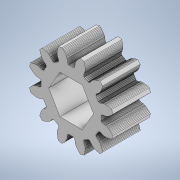
# Autodesk Inventor part: Engranajes_12
Saved by Autodesk Inventor 2022 (Build 260153000, 153)
## iProperties
Created: 2022-02-21
Part Number: Engranajes_12
Material: Generic
Document SubType Name: Modeling
Designer: katha
Density: 1 g/cm^3
Appearance: Default
Author: katha
Autodesk Inventor part; units mm, degrees
(part 1 of 6)
ref_plane "YZ Plane" through (0, 0, 0) normal (1, 0, 0) x (0, 1, 0)
ref_plane "XZ Plane" through (0, 0, 0) normal (0, 1, 0) x (-1, 0, 0)
ref_plane "XY Plane" through (0, 0, 0) normal (0, 0, 1) x (1, 0, 0)
sketch "Sketch1" plane through (0, 0, 0) normal (0, 0, 1) x (1, 0, 0)
  circle A0 centre (36, 0) radius 2
  circle A1 centre (0, 0) radius 2
  circle A2 centre (36, 0) radius 2
  circle A3 centre (0, 0) radius 2
  line L0 (30.8694, -4.5708) -> (30.9098, -4.4161)
  line L1 (30.9098, -4.4161) -> (30.9538, -4.2725)
  line L2 (30.9538, -4.2725) -> (31.0003, -4.1408)
  line L3 (31.0003, -4.1408) -> (31.0488, -4.0198)
  line L4 (31.0488, -4.0198) -> (31.0977, -3.9112)
  line L5 (31.0977, -3.9112) -> (31.1475, -3.8119)
  line L6 (31.1475, -3.8119) -> (31.1956, -3.7252)
  line L7 (31.1956, -3.7252) -> (31.2429, -3.6478)
  line L8 (31.2429, -3.6478) -> (31.2875, -3.5813)
  line L9 (31.2875, -3.5813) -> (31.3671, -3.477)
  line L10 (31.3671, -3.477) -> (31.4285, -3.4089)
  line L11 (31.4285, -3.4089) -> (31.466, -3.3746)
  line L12 (31.466, -3.3746) -> (31.5668, -3.3141)
  line L13 (31.5668, -3.3141) -> (31.6547, -3.2516)
  line L14 (31.6547, -3.2516) -> (31.7296, -3.1879)
  line L15 (31.7296, -3.1879) -> (31.7917, -3.1241)
  line L16 (31.7917, -3.1241) -> (31.841, -3.0611)
  line L17 (31.841, -3.0611) -> (31.8779, -2.9999)
  line L18 (31.8779, -2.9999) -> (31.9025, -2.9414)
  line L19 (31.9025, -2.9414) -> (31.9152, -2.8864)
  line L20 (31.9152, -2.8864) -> (31.9163, -2.836)
  line L21 (31.9163, -2.836) -> (31.9062, -2.7909)
  line L22 (31.9062, -2.7909) -> (31.8916, -2.7611)
  line L23 (31.8916, -2.7611) -> (31.8003, -2.6202)
  line L24 (31.8003, -2.6202) -> (31.7132, -2.475)
  line L25 (31.7132, -2.475) -> (31.631, -2.327)
  line L26 (31.631, -2.327) -> (31.5546, -2.1774)
  line L27 (31.5546, -2.1774) -> (31.5361, -2.1499)
  line L28 (31.5361, -2.1499) -> (31.5021, -2.1186)
  line L29 (31.5021, -2.1186) -> (31.4579, -2.0943)
  line L30 (31.4579, -2.0943) -> (31.404, -2.0778)
  line L31 (31.404, -2.0778) -> (31.341, -2.0699)
  line L32 (31.341, -2.0699) -> (31.2695, -2.0712)
  line L33 (31.2695, -2.0712) -> (31.1903, -2.0825)
  line L34 (31.1903, -2.0825) -> (31.104, -2.1043)
  line L35 (31.104, -2.1043) -> (31.0114, -2.1374)
  line L36 (31.0114, -2.1374) -> (30.9133, -2.1822)
  line L37 (30.9133, -2.1822) -> (30.8106, -2.2393)
  line L38 (30.8106, -2.2393) -> (30.762, -2.2546)
  line L39 (30.762, -2.2546) -> (30.6724, -2.2738)
  line L40 (30.6724, -2.2738) -> (30.5422, -2.2905)
  line L41 (30.5422, -2.2905) -> (30.4624, -2.2959)
  line L42 (30.4624, -2.2959) -> (30.3717, -2.2981)
  line L43 (30.3717, -2.2981) -> (30.2725, -2.2965)
  line L44 (30.2725, -2.2965) -> (30.1616, -2.2899)
  line L45 (30.1616, -2.2899) -> (30.0431, -2.278)
  line L46 (30.0431, -2.278) -> (29.9141, -2.2595)
  line L47 (29.9141, -2.2595) -> (29.7768, -2.2339)
  line L48 (29.7768, -2.2339) -> (29.6305, -2.2002)
  line L49 (29.6305, -2.2002) -> (29.4762, -2.1578)
  line L50 (29.4762, -2.1578) -> (29.3255, -2.1096)
  arc A4 (29.1649, -1.5103) -> (29.3255, -2.1096) centre (36, 0) ccw
  line L51 (29.1649, -1.5103) -> (29.2713, -1.3932)
  line L52 (29.2713, -1.3932) -> (29.3837, -1.2793)
  line L53 (29.3837, -1.2793) -> (29.4936, -1.177)
  line L54 (29.4936, -1.177) -> (29.5997, -1.0861)
  line L55 (29.5997, -1.0861) -> (29.7022, -1.0056)
  line L56 (29.7022, -1.0056) -> (29.7988, -0.9361)
  line L57 (29.7988, -0.9361) -> (29.8916, -0.875)
  line L58 (29.8916, -0.875) -> (29.9767, -0.8239)
  line L59 (29.9767, -0.8239) -> (30.0563, -0.7805)
  line L60 (30.0563, -0.7805) -> (30.1282, -0.7452)
  line L61 (30.1282, -0.7452) -> (30.2493, -0.6947)
  line L62 (30.2493, -0.6947) -> (30.3365, -0.6665)
  line L63 (30.3365, -0.6665) -> (30.3862, -0.6555)
  line L64 (30.3862, -0.6555) -> (30.5037, -0.6535)
  line L65 (30.5037, -0.6535) -> (30.611, -0.6433)
  line L66 (30.611, -0.6433) -> (30.7078, -0.6256)
  line L67 (30.7078, -0.6256) -> (30.7934, -0.6014)
  line L68 (30.7934, -0.6014) -> (30.8677, -0.5716)
  line L69 (30.8677, -0.5716) -> (30.9302, -0.537)
  line L70 (30.9302, -0.537) -> (30.9808, -0.4986)
  line L71 (30.9808, -0.4986) -> (31.0192, -0.4573)
  line L72 (31.0192, -0.4573) -> (31.0454, -0.4142)
  line L73 (31.0454, -0.4142) -> (31.0592, -0.3701)
  line L74 (31.0592, -0.3701) -> (31.0614, -0.337)
  line L75 (31.0614, -0.337) -> (31.0529, -0.1693)
  line L76 (31.0529, -0.1693) -> (31.05, 0)
  line L77 (31.05, 0) -> (31.0529, 0.1693)
  line L78 (31.0529, 0.1693) -> (31.0614, 0.337)
  line L79 (31.0614, 0.337) -> (31.0592, 0.3701)
  line L80 (31.0592, 0.3701) -> (31.0454, 0.4142)
  line L81 (31.0454, 0.4142) -> (31.0192, 0.4573)
  line L82 (31.0192, 0.4573) -> (30.9808, 0.4986)
  line L83 (30.9808, 0.4986) -> (30.9302, 0.537)
  line L84 (30.9302, 0.537) -> (30.8677, 0.5716)
  line L85 (30.8677, 0.5716) -> (30.7934, 0.6014)
  line L86 (30.7934, 0.6014) -> (30.7078, 0.6256)
  line L87 (30.7078, 0.6256) -> (30.611, 0.6433)
  line L88 (30.611, 0.6433) -> (30.5037, 0.6535)
  line L89 (30.5037, 0.6535) -> (30.3862, 0.6555)
  line L90 (30.3862, 0.6555) -> (30.3365, 0.6665)
  line L91 (30.3365, 0.6665) -> (30.2493, 0.6947)
  line L92 (30.2493, 0.6947) -> (30.1282, 0.7452)
  line L93 (30.1282, 0.7452) -> (30.0563, 0.7805)
  line L94 (30.0563, 0.7805) -> (29.9767, 0.8239)
  line L95 (29.9767, 0.8239) -> (29.8916, 0.875)
  line L96 (29.8916, 0.875) -> (29.7988, 0.9361)
  line L97 (29.7988, 0.9361) -> (29.7022, 1.0056)
  line L98 (29.7022, 1.0056) -> (29.5997, 1.0861)
  line L99 (29.5997, 1.0861) -> (29.4936, 1.177)
  line L100 (29.4936, 1.177) -> (29.3837, 1.2793)
  line L101 (29.3837, 1.2793) -> (29.2713, 1.3932)
  line L102 (29.2713, 1.3932) -> (29.1649, 1.5103)
  arc A5 (29.3255, 2.1096) -> (29.1649, 1.5103) centre (36, 0) ccw
  line L103 (29.3255, 2.1096) -> (29.4762, 2.1578)
  line L104 (29.4762, 2.1578) -> (29.6305, 2.2002)
  line L105 (29.6305, 2.2002) -> (29.7768, 2.2339)
  line L106 (29.7768, 2.2339) -> (29.9141, 2.2595)
  line L107 (29.9141, 2.2595) -> (30.0431, 2.278)
  line L108 (30.0431, 2.278) -> (30.1616, 2.2899)
  line L109 (30.1616, 2.2899) -> (30.2725, 2.2965)
  line L110 (30.2725, 2.2965) -> (30.3717, 2.2981)
  line L111 (30.3717, 2.2981) -> (30.4624, 2.2959)
  line L112 (30.4624, 2.2959) -> (30.5422, 2.2905)
  line L113 (30.5422, 2.2905) -> (30.6724, 2.2738)
  line L114 (30.6724, 2.2738) -> (30.762, 2.2546)
  line L115 (30.762, 2.2546) -> (30.8106, 2.2393)
  line L116 (30.8106, 2.2393) -> (30.9133, 2.1822)
  line L117 (30.9133, 2.1822) -> (31.0114, 2.1374)
  line L118 (31.0114, 2.1374) -> (31.104, 2.1043)
  line L119 (31.104, 2.1043) -> (31.1903, 2.0825)
  line L120 (31.1903, 2.0825) -> (31.2695, 2.0712)
  line L121 (31.2695, 2.0712) -> (31.341, 2.0699)
  line L122 (31.341, 2.0699) -> (31.404, 2.0778)
  line L123 (31.404, 2.0778) -> (31.4579, 2.0943)
  line L124 (31.4579, 2.0943) -> (31.5021, 2.1186)
  line L125 (31.5021, 2.1186) -> (31.5361, 2.1499)
  line L126 (31.5361, 2.1499) -> (31.5546, 2.1774)
  line L127 (31.5546, 2.1774) -> (31.631, 2.327)
  line L128 (31.631, 2.327) -> (31.7132, 2.475)
  line L129 (31.7132, 2.475) -> (31.8003, 2.6202)
  line L130 (31.8003, 2.6202) -> (31.8916, 2.7611)
  line L131 (31.8916, 2.7611) -> (31.9062, 2.7909)
  line L132 (31.9062, 2.7909) -> (31.9163, 2.836)
  line L133 (31.9163, 2.836) -> (31.9152, 2.8864)
  line L134 (31.9152, 2.8864) -> (31.9025, 2.9414)
  line L135 (31.9025, 2.9414) -> (31.8779, 2.9999)
  line L136 (31.8779, 2.9999) -> (31.841, 3.0611)
  line L137 (31.841, 3.0611) -> (31.7917, 3.1241)
  line L138 (31.7917, 3.1241) -> (31.7296, 3.1879)
  line L139 (31.7296, 3.1879) -> (31.6547, 3.2516)
  line L140 (31.6547, 3.2516) -> (31.5668, 3.3141)
  line L141 (31.5668, 3.3141) -> (31.466, 3.3746)
  line L142 (31.466, 3.3746) -> (31.4285, 3.4089)
  line L143 (31.4285, 3.4089) -> (31.3671, 3.477)
  line L144 (31.3671, 3.477) -> (31.2875, 3.5813)
  line L145 (31.2875, 3.5813) -> (31.2429, 3.6478)
  line L146 (31.2429, 3.6478) -> (31.1956, 3.7252)
  line L147 (31.1956, 3.7252) -> (31.1475, 3.8119)
  line L148 (31.1475, 3.8119) -> (31.0977, 3.9112)
  line L149 (31.0977, 3.9112) -> (31.0488, 4.0198)
  line L150 (31.0488, 4.0198) -> (31.0003, 4.1408)
  line L151 (31.0003, 4.1408) -> (30.9538, 4.2725)
  line L152 (30.9538, 4.2725) -> (30.9098, 4.4161)
  line L153 (30.9098, 4.4161) -> (30.8694, 4.5708)
  line L154 (30.8694, 4.5708) -> (30.8358, 4.7255)
  arc A6 (31.2745, 5.1642) -> (30.8358, 4.7255) centre (36, 0) ccw
  line L155 (31.2745, 5.1642) -> (31.4292, 5.1306)
  line L156 (31.4292, 5.1306) -> (31.5839, 5.0902)
  line L157 (31.5839, 5.0902) -> (31.7275, 5.0462)
  line L158 (31.7275, 5.0462) -> (31.8592, 4.9997)
  line L159 (31.8592, 4.9997) -> (31.9802, 4.9512)
  line L160 (31.9802, 4.9512) -> (32.0888, 4.9023)
  line L161 (32.0888, 4.9023) -> (32.1881, 4.8525)
  line L162 (32.1881, 4.8525) -> (32.2748, 4.8044)
  line L163 (32.2748, 4.8044) -> (32.3522, 4.7571)
  line L164 (32.3522, 4.7571) -> (32.4187, 4.7125)
  line L165 (32.4187, 4.7125) -> (32.523, 4.6329)
  line L166 (32.523, 4.6329) -> (32.5911, 4.5715)
  line L167 (32.5911, 4.5715) -> (32.6254, 4.534)
  line L168 (32.6254, 4.534) -> (32.6859, 4.4332)
  line L169 (32.6859, 4.4332) -> (32.7484, 4.3453)
  line L170 (32.7484, 4.3453) -> (32.8121, 4.2704)
  line L171 (32.8121, 4.2704) -> (32.8759, 4.2083)
  line L172 (32.8759, 4.2083) -> (32.9389, 4.159)
  line L173 (32.9389, 4.159) -> (33.0001, 4.1221)
  line L174 (33.0001, 4.1221) -> (33.0586, 4.0975)
  line L175 (33.0586, 4.0975) -> (33.1136, 4.0848)
  line L176 (33.1136, 4.0848) -> (33.164, 4.0837)
  line L177 (33.164, 4.0837) -> (33.2091, 4.0938)
  line L178 (33.2091, 4.0938) -> (33.2389, 4.1084)
  line L179 (33.2389, 4.1084) -> (33.3798, 4.1997)
  line L180 (33.3798, 4.1997) -> (33.525, 4.2868)
  line L181 (33.525, 4.2868) -> (33.673, 4.369)
  line L182 (33.673, 4.369) -> (33.8226, 4.4454)
  line L183 (33.8226, 4.4454) -> (33.8501, 4.4639)
  line L184 (33.8501, 4.4639) -> (33.8814, 4.4979)
  line L185 (33.8814, 4.4979) -> (33.9057, 4.5421)
  line L186 (33.9057, 4.5421) -> (33.9222, 4.596)
  line L187 (33.9222, 4.596) -> (33.9301, 4.659)
  line L188 (33.9301, 4.659) -> (33.9288, 4.7305)
  line L189 (33.9288, 4.7305) -> (33.9175, 4.8097)
  line L190 (33.9175, 4.8097) -> (33.8957, 4.896)
  line L191 (33.8957, 4.896) -> (33.8626, 4.9886)
  line L192 (33.8626, 4.9886) -> (33.8178, 5.0867)
  line L193 (33.8178, 5.0867) -> (33.7607, 5.1894)
  line L194 (33.7607, 5.1894) -> (33.7454, 5.238)
  line L195 (33.7454, 5.238) -> (33.7262, 5.3276)
  line L196 (33.7262, 5.3276) -> (33.7095, 5.4578)
  line L197 (33.7095, 5.4578) -> (33.7041, 5.5376)
  line L198 (33.7041, 5.5376) -> (33.7019, 5.6283)
  line L199 (33.7019, 5.6283) -> (33.7035, 5.7275)
  line L200 (33.7035, 5.7275) -> (33.7101, 5.8384)
  line L201 (33.7101, 5.8384) -> (33.722, 5.9569)
  line L202 (33.722, 5.9569) -> (33.7405, 6.0859)
  line L203 (33.7405, 6.0859) -> (33.7661, 6.2232)
  line L204 (33.7661, 6.2232) -> (33.7998, 6.3695)
  line L205 (33.7998, 6.3695) -> (33.8422, 6.5238)
  line L206 (33.8422, 6.5238) -> (33.8904, 6.6745)
  arc A7 (34.4897, 6.8351) -> (33.8904, 6.6745) centre (36, 0) ccw
  line L207 (34.4897, 6.8351) -> (34.6069, 6.7287)
  line L208 (34.6069, 6.7287) -> (34.7207, 6.6163)
  line L209 (34.7207, 6.6163) -> (34.823, 6.5064)
  line L210 (34.823, 6.5064) -> (34.9138, 6.4003)
  line L211 (34.9138, 6.4003) -> (34.9944, 6.2978)
  line L212 (34.9944, 6.2978) -> (35.0639, 6.2012)
  line L213 (35.0639, 6.2012) -> (35.125, 6.1084)
  line L214 (35.125, 6.1084) -> (35.1761, 6.0233)
  line L215 (35.1761, 6.0233) -> (35.2195, 5.9436)
  line L216 (35.2195, 5.9436) -> (35.2548, 5.8718)
  line L217 (35.2548, 5.8718) -> (35.3053, 5.7507)
  line L218 (35.3053, 5.7507) -> (35.3335, 5.6635)
  line L219 (35.3335, 5.6635) -> (35.3445, 5.6138)
  line L220 (35.3445, 5.6138) -> (35.3465, 5.4963)
  line L221 (35.3465, 5.4963) -> (35.3567, 5.389)
  line L222 (35.3567, 5.389) -> (35.3744, 5.2923)
  line L223 (35.3744, 5.2923) -> (35.3986, 5.2066)
  line L224 (35.3986, 5.2066) -> (35.4284, 5.1323)
  line L225 (35.4284, 5.1323) -> (35.463, 5.0698)
  line L226 (35.463, 5.0698) -> (35.5014, 5.0192)
  line L227 (35.5014, 5.0192) -> (35.5427, 4.9808)
  line L228 (35.5427, 4.9808) -> (35.5858, 4.9546)
  line L229 (35.5858, 4.9546) -> (35.6299, 4.9408)
  line L230 (35.6299, 4.9408) -> (35.663, 4.9386)
  line L231 (35.663, 4.9386) -> (35.8307, 4.9471)
  line L232 (35.8307, 4.9471) -> (36, 4.95)
  line L233 (36, 4.95) -> (36.1693, 4.9471)
  line L234 (36.1693, 4.9471) -> (36.337, 4.9386)
  line L235 (36.337, 4.9386) -> (36.3701, 4.9408)
  line L236 (36.3701, 4.9408) -> (36.4142, 4.9546)
  line L237 (36.4142, 4.9546) -> (36.4573, 4.9808)
  line L238 (36.4573, 4.9808) -> (36.4986, 5.0192)
  line L239 (36.4986, 5.0192) -> (36.537, 5.0698)
  line L240 (36.537, 5.0698) -> (36.5716, 5.1323)
  line L241 (36.5716, 5.1323) -> (36.6014, 5.2066)
  line L242 (36.6014, 5.2066) -> (36.6256, 5.2923)
  line L243 (36.6256, 5.2923) -> (36.6433, 5.389)
  line L244 (36.6433, 5.389) -> (36.6535, 5.4963)
  line L245 (36.6535, 5.4963) -> (36.6555, 5.6138)
  line L246 (36.6555, 5.6138) -> (36.6665, 5.6635)
  line L247 (36.6665, 5.6635) -> (36.6947, 5.7507)
  line L248 (36.6947, 5.7507) -> (36.7452, 5.8718)
  line L249 (36.7452, 5.8718) -> (36.7805, 5.9436)
  line L250 (36.7805, 5.9436) -> (36.8239, 6.0233)
  line L251 (36.8239, 6.0233) -> (36.875, 6.1084)
  line L252 (36.875, 6.1084) -> (36.9361, 6.2012)
  line L253 (36.9361, 6.2012) -> (37.0056, 6.2978)
  line L254 (37.0056, 6.2978) -> (37.0862, 6.4003)
  line L255 (37.0862, 6.4003) -> (37.177, 6.5064)
  line L256 (37.177, 6.5064) -> (37.2793, 6.6163)
  line L257 (37.2793, 6.6163) -> (37.3931, 6.7287)
  line L258 (37.3931, 6.7287) -> (37.5103, 6.8351)
  arc A8 (38.1096, 6.6745) -> (37.5103, 6.8351) centre (36, 0) ccw
  line L259 (38.1096, 6.6745) -> (38.1578, 6.5238)
  line L260 (38.1578, 6.5238) -> (38.2002, 6.3695)
  line L261 (38.2002, 6.3695) -> (38.2339, 6.2232)
  line L262 (38.2339, 6.2232) -> (38.2595, 6.0859)
  line L263 (38.2595, 6.0859) -> (38.278, 5.9569)
  line L264 (38.278, 5.9569) -> (38.2899, 5.8384)
  line L265 (38.2899, 5.8384) -> (38.2965, 5.7275)
  line L266 (38.2965, 5.7275) -> (38.2981, 5.6283)
  line L267 (38.2981, 5.6283) -> (38.2959, 5.5376)
  line L268 (38.2959, 5.5376) -> (38.2905, 5.4578)
  line L269 (38.2905, 5.4578) -> (38.2738, 5.3276)
  line L270 (38.2738, 5.3276) -> (38.2546, 5.238)
  line L271 (38.2546, 5.238) -> (38.2393, 5.1894)
  line L272 (38.2393, 5.1894) -> (38.1822, 5.0867)
  line L273 (38.1822, 5.0867) -> (38.1374, 4.9886)
  line L274 (38.1374, 4.9886) -> (38.1043, 4.896)
  line L275 (38.1043, 4.896) -> (38.0825, 4.8097)
  line L276 (38.0825, 4.8097) -> (38.0712, 4.7305)
  line L277 (38.0712, 4.7305) -> (38.0699, 4.659)
  line L278 (38.0699, 4.659) -> (38.0778, 4.596)
  line L279 (38.0778, 4.596) -> (38.0943, 4.5421)
  line L280 (38.0943, 4.5421) -> (38.1186, 4.4979)
  line L281 (38.1186, 4.4979) -> (38.1499, 4.4639)
  line L282 (38.1499, 4.4639) -> (38.1774, 4.4454)
  line L283 (38.1774, 4.4454) -> (38.327, 4.369)
  line L284 (38.327, 4.369) -> (38.475, 4.2868)
  line L285 (38.475, 4.2868) -> (38.6202, 4.1997)
  line L286 (38.6202, 4.1997) -> (38.7611, 4.1084)
  line L287 (38.7611, 4.1084) -> (38.7909, 4.0938)
  line L288 (38.7909, 4.0938) -> (38.836, 4.0837)
  line L289 (38.836, 4.0837) -> (38.8864, 4.0848)
  line L290 (38.8864, 4.0848) -> (38.9414, 4.0975)
  line L291 (38.9414, 4.0975) -> (38.9999, 4.1221)
  line L292 (38.9999, 4.1221) -> (39.0611, 4.159)
  line L293 (39.0611, 4.159) -> (39.1241, 4.2083)
  line L294 (39.1241, 4.2083) -> (39.1879, 4.2704)
  line L295 (39.1879, 4.2704) -> (39.2516, 4.3453)
  line L296 (39.2516, 4.3453) -> (39.3141, 4.4332)
  line L297 (39.3141, 4.4332) -> (39.3746, 4.534)
  line L298 (39.3746, 4.534) -> (39.4089, 4.5715)
  line L299 (39.4089, 4.5715) -> (39.477, 4.6329)
  line L300 (39.477, 4.6329) -> (39.5813, 4.7125)
  line L301 (39.5813, 4.7125) -> (39.6478, 4.7571)
  line L302 (39.6478, 4.7571) -> (39.7252, 4.8044)
  line L303 (39.7252, 4.8044) -> (39.8119, 4.8525)
  line L304 (39.8119, 4.8525) -> (39.9112, 4.9023)
  line L305 (39.9112, 4.9023) -> (40.0198, 4.9512)
  line L306 (40.0198, 4.9512) -> (40.1408, 4.9997)
  line L307 (40.1408, 4.9997) -> (40.2725, 5.0462)
  line L308 (40.2725, 5.0462) -> (40.4161, 5.0902)
  line L309 (40.4161, 5.0902) -> (40.5708, 5.1306)
  line L310 (40.5708, 5.1306) -> (40.7255, 5.1642)
  arc A9 (41.1642, 4.7255) -> (40.7255, 5.1642) centre (36, 0) ccw
  line L311 (41.1642, 4.7255) -> (41.1306, 4.5708)
  line L312 (41.1306, 4.5708) -> (41.0902, 4.4161)
  line L313 (41.0902, 4.4161) -> (41.0462, 4.2725)
  line L314 (41.0462, 4.2725) -> (40.9997, 4.1408)
  line L315 (40.9997, 4.1408) -> (40.9512, 4.0198)
  line L316 (40.9512, 4.0198) -> (40.9023, 3.9112)
  line L317 (40.9023, 3.9112) -> (40.8525, 3.8119)
  line L318 (40.8525, 3.8119) -> (40.8044, 3.7252)
  line L319 (40.8044, 3.7252) -> (40.7571, 3.6478)
  line L320 (40.7571, 3.6478) -> (40.7125, 3.5813)
  line L321 (40.7125, 3.5813) -> (40.6329, 3.477)
  line L322 (40.6329, 3.477) -> (40.5715, 3.4089)
  line L323 (40.5715, 3.4089) -> (40.534, 3.3746)
  line L324 (40.534, 3.3746) -> (40.4332, 3.3141)
  line L325 (40.4332, 3.3141) -> (40.3453, 3.2516)
  line L326 (40.3453, 3.2516) -> (40.2704, 3.1879)
  line L327 (40.2704, 3.1879) -> (40.2083, 3.1241)
  line L328 (40.2083, 3.1241) -> (40.159, 3.0611)
  line L329 (40.159, 3.0611) -> (40.1221, 2.9999)
  line L330 (40.1221, 2.9999) -> (40.0975, 2.9414)
  line L331 (40.0975, 2.9414) -> (40.0848, 2.8864)
  line L332 (40.0848, 2.8864) -> (40.0837, 2.836)
  line L333 (40.0837, 2.836) -> (40.0938, 2.7909)
  line L334 (40.0938, 2.7909) -> (40.1084, 2.7611)
  line L335 (40.1084, 2.7611) -> (40.1997, 2.6202)
  line L336 (40.1997, 2.6202) -> (40.2868, 2.475)
  line L337 (40.2868, 2.475) -> (40.369, 2.327)
  line L338 (40.369, 2.327) -> (40.4454, 2.1774)
  line L339 (40.4454, 2.1774) -> (40.4639, 2.1499)
  line L340 (40.4639, 2.1499) -> (40.4979, 2.1186)
  line L341 (40.4979, 2.1186) -> (40.5421, 2.0943)
  line L342 (40.5421, 2.0943) -> (40.596, 2.0778)
  line L343 (40.596, 2.0778) -> (40.659, 2.0699)
  line L344 (40.659, 2.0699) -> (40.7305, 2.0712)
  line L345 (40.7305, 2.0712) -> (40.8097, 2.0825)
  line L346 (40.8097, 2.0825) -> (40.896, 2.1043)
  line L347 (40.896, 2.1043) -> (40.9886, 2.1374)
  line L348 (40.9886, 2.1374) -> (41.0867, 2.1822)
  line L349 (41.0867, 2.1822) -> (41.1894, 2.2393)
  line L350 (41.1894, 2.2393) -> (41.238, 2.2546)
  line L351 (41.238, 2.2546) -> (41.3276, 2.2738)
  line L352 (41.3276, 2.2738) -> (41.4578, 2.2905)
  line L353 (41.4578, 2.2905) -> (41.5376, 2.2959)
  line L354 (41.5376, 2.2959) -> (41.6283, 2.2981)
  line L355 (41.6283, 2.2981) -> (41.7275, 2.2965)
  line L356 (41.7275, 2.2965) -> (41.8384, 2.2899)
  line L357 (41.8384, 2.2899) -> (41.9569, 2.278)
  line L358 (41.9569, 2.278) -> (42.0859, 2.2595)
  line L359 (42.0859, 2.2595) -> (42.2232, 2.2339)
  line L360 (42.2232, 2.2339) -> (42.3695, 2.2002)
  line L361 (42.3695, 2.2002) -> (42.5238, 2.1578)
  line L362 (42.5238, 2.1578) -> (42.6745, 2.1096)
  arc A10 (42.8351, 1.5103) -> (42.6745, 2.1096) centre (36, 0) ccw
  line L363 (42.8351, 1.5103) -> (42.7287, 1.3932)
  line L364 (42.7287, 1.3932) -> (42.6163, 1.2793)
  line L365 (42.6163, 1.2793) -> (42.5064, 1.177)
  line L366 (42.5064, 1.177) -> (42.4003, 1.0861)
  line L367 (42.4003, 1.0861) -> (42.2978, 1.0056)
  line L368 (42.2978, 1.0056) -> (42.2012, 0.9361)
  line L369 (42.2012, 0.9361) -> (42.1084, 0.875)
  line L370 (42.1084, 0.875) -> (42.0233, 0.8239)
  line L371 (42.0233, 0.8239) -> (41.9437, 0.7805)
  line L372 (41.9437, 0.7805) -> (41.8718, 0.7452)
  line L373 (41.8718, 0.7452) -> (41.7507, 0.6947)
  line L374 (41.7507, 0.6947) -> (41.6635, 0.6665)
  line L375 (41.6635, 0.6665) -> (41.6138, 0.6555)
  line L376 (41.6138, 0.6555) -> (41.4963, 0.6535)
  line L377 (41.4963, 0.6535) -> (41.389, 0.6433)
  line L378 (41.389, 0.6433) -> (41.2923, 0.6256)
  line L379 (41.2923, 0.6256) -> (41.2066, 0.6014)
  line L380 (41.2066, 0.6014) -> (41.1323, 0.5716)
  line L381 (41.1323, 0.5716) -> (41.0698, 0.537)
  line L382 (41.0698, 0.537) -> (41.0192, 0.4986)
  line L383 (41.0192, 0.4986) -> (40.9808, 0.4573)
  line L384 (40.9808, 0.4573) -> (40.9546, 0.4142)
  line L385 (40.9546, 0.4142) -> (40.9408, 0.3701)
  line L386 (40.9408, 0.3701) -> (40.9386, 0.337)
  line L387 (40.9386, 0.337) -> (40.9471, 0.1693)
  line L388 (40.9471, 0.1693) -> (40.95, 0)
  line L389 (40.95, 0) -> (40.9471, -0.1693)
  line L390 (40.9471, -0.1693) -> (40.9386, -0.337)
  line L391 (40.9386, -0.337) -> (40.9408, -0.3701)
  line L392 (40.9408, -0.3701) -> (40.9546, -0.4142)
  line L393 (40.9546, -0.4142) -> (40.9808, -0.4573)
  line L394 (40.9808, -0.4573) -> (41.0192, -0.4986)
  line L395 (41.0192, -0.4986) -> (41.0698, -0.537)
  line L396 (41.0698, -0.537) -> (41.1323, -0.5716)
  line L397 (41.1323, -0.5716) -> (41.2066, -0.6014)
  line L398 (41.2066, -0.6014) -> (41.2923, -0.6256)
  line L399 (41.2923, -0.6256) -> (41.389, -0.6433)
  line L400 (41.389, -0.6433) -> (41.4963, -0.6535)
  line L401 (41.4963, -0.6535) -> (41.6138, -0.6555)
  line L402 (41.6138, -0.6555) -> (41.6635, -0.6665)
  line L403 (41.6635, -0.6665) -> (41.7507, -0.6947)
  line L404 (41.7507, -0.6947) -> (41.8718, -0.7452)
  line L405 (41.8718, -0.7452) -> (41.9437, -0.7805)
  line L406 (41.9437, -0.7805) -> (42.0233, -0.8239)
  line L407 (42.0233, -0.8239) -> (42.1084, -0.875)
  line L408 (42.1084, -0.875) -> (42.2012, -0.9361)
  line L409 (42.2012, -0.9361) -> (42.2978, -1.0056)
  line L410 (42.2978, -1.0056) -> (42.4003, -1.0861)
  line L411 (42.4003, -1.0861) -> (42.5064, -1.177)
  line L412 (42.5064, -1.177) -> (42.6163, -1.2793)
  line L413 (42.6163, -1.2793) -> (42.7287, -1.3932)
  line L414 (42.7287, -1.3932) -> (42.8351, -1.5103)
  arc A11 (42.6745, -2.1096) -> (42.8351, -1.5103) centre (36, 0) ccw
  line L415 (42.6745, -2.1096) -> (42.5238, -2.1578)
  line L416 (42.5238, -2.1578) -> (42.3695, -2.2002)
  line L417 (42.3695, -2.2002) -> (42.2232, -2.2339)
  line L418 (42.2232, -2.2339) -> (42.0859, -2.2595)
  line L419 (42.0859, -2.2595) -> (41.9569, -2.278)
  line L420 (41.9569, -2.278) -> (41.8384, -2.2899)
  line L421 (41.8384, -2.2899) -> (41.7275, -2.2965)
  line L422 (41.7275, -2.2965) -> (41.6283, -2.2981)
  line L423 (41.6283, -2.2981) -> (41.5376, -2.2959)
  line L424 (41.5376, -2.2959) -> (41.4578, -2.2905)
  line L425 (41.4578, -2.2905) -> (41.3276, -2.2738)
  line L426 (41.3276, -2.2738) -> (41.238, -2.2546)
  line L427 (41.238, -2.2546) -> (41.1894, -2.2393)
  line L428 (41.1894, -2.2393) -> (41.0867, -2.1822)
  line L429 (41.0867, -2.1822) -> (40.9886, -2.1374)
  line L430 (40.9886, -2.1374) -> (40.896, -2.1043)
  line L431 (40.896, -2.1043) -> (40.8097, -2.0825)
  line L432 (40.8097, -2.0825) -> (40.7305, -2.0712)
  line L433 (40.7305, -2.0712) -> (40.659, -2.0699)
  line L434 (40.659, -2.0699) -> (40.596, -2.0778)
  line L435 (40.596, -2.0778) -> (40.5421, -2.0943)
  line L436 (40.5421, -2.0943) -> (40.4979, -2.1186)
  line L437 (40.4979, -2.1186) -> (40.4639, -2.1499)
  line L438 (40.4639, -2.1499) -> (40.4454, -2.1774)
  line L439 (40.4454, -2.1774) -> (40.369, -2.327)
  line L440 (40.369, -2.327) -> (40.2868, -2.475)
  line L441 (40.2868, -2.475) -> (40.1997, -2.6202)
  line L442 (40.1997, -2.6202) -> (40.1084, -2.7611)
  line L443 (40.1084, -2.7611) -> (40.0938, -2.7909)
  line L444 (40.0938, -2.7909) -> (40.0837, -2.836)
  line L445 (40.0837, -2.836) -> (40.0848, -2.8864)
  line L446 (40.0848, -2.8864) -> (40.0975, -2.9414)
  line L447 (40.0975, -2.9414) -> (40.1221, -2.9999)
  line L448 (40.1221, -2.9999) -> (40.159, -3.0611)
  line L449 (40.159, -3.0611) -> (40.2083, -3.1241)
  line L450 (40.2083, -3.1241) -> (40.2704, -3.1879)
  line L451 (40.2704, -3.1879) -> (40.3453, -3.2516)
  line L452 (40.3453, -3.2516) -> (40.4332, -3.3141)
  line L453 (40.4332, -3.3141) -> (40.534, -3.3746)
  line L454 (40.534, -3.3746) -> (40.5715, -3.4089)
  line L455 (40.5715, -3.4089) -> (40.6329, -3.477)
  line L456 (40.6329, -3.477) -> (40.7125, -3.5813)
  line L457 (40.7125, -3.5813) -> (40.7571, -3.6478)
  line L458 (40.7571, -3.6478) -> (40.8044, -3.7252)
  line L459 (40.8044, -3.7252) -> (40.8525, -3.8119)
  line L460 (40.8525, -3.8119) -> (40.9023, -3.9112)
  line L461 (40.9023, -3.9112) -> (40.9512, -4.0198)
  line L462 (40.9512, -4.0198) -> (40.9997, -4.1408)
  line L463 (40.9997, -4.1408) -> (41.0462, -4.2725)
  line L464 (41.0462, -4.2725) -> (41.0902, -4.4161)
  line L465 (41.0902, -4.4161) -> (41.1306, -4.5708)
  line L466 (41.1306, -4.5708) -> (41.1642, -4.7255)
  arc A12 (40.7255, -5.1642) -> (41.1642, -4.7255) centre (36, 0) ccw
  line L467 (40.7255, -5.1642) -> (40.5708, -5.1306)
  line L468 (40.5708, -5.1306) -> (40.4161, -5.0902)
  line L469 (40.4161, -5.0902) -> (40.2725, -5.0462)
  line L470 (40.2725, -5.0462) -> (40.1408, -4.9997)
  line L471 (40.1408, -4.9997) -> (40.0198, -4.9512)
  line L472 (40.0198, -4.9512) -> (39.9112, -4.9023)
  line L473 (39.9112, -4.9023) -> (39.8119, -4.8525)
  line L474 (39.8119, -4.8525) -> (39.7252, -4.8044)
  line L475 (39.7252, -4.8044) -> (39.6478, -4.7571)
  line L476 (39.6478, -4.7571) -> (39.5813, -4.7125)
  line L477 (39.5813, -4.7125) -> (39.477, -4.6329)
  line L478 (39.477, -4.6329) -> (39.4089, -4.5715)
  line L479 (39.4089, -4.5715) -> (39.3746, -4.534)
  line L480 (39.3746, -4.534) -> (39.3141, -4.4332)
  line L481 (39.3141, -4.4332) -> (39.2516, -4.3453)
  line L482 (39.2516, -4.3453) -> (39.1879, -4.2704)
  line L483 (39.1879, -4.2704) -> (39.1241, -4.2083)
  line L484 (39.1241, -4.2083) -> (39.0611, -4.159)
  line L485 (39.0611, -4.159) -> (38.9999, -4.1221)
  line L486 (38.9999, -4.1221) -> (38.9414, -4.0975)
  line L487 (38.9414, -4.0975) -> (38.8864, -4.0848)
  line L488 (38.8864, -4.0848) -> (38.836, -4.0837)
  line L489 (38.836, -4.0837) -> (38.7909, -4.0938)
  line L490 (38.7909, -4.0938) -> (38.7611, -4.1084)
  line L491 (38.7611, -4.1084) -> (38.6202, -4.1997)
  line L492 (38.6202, -4.1997) -> (38.475, -4.2868)
  line L493 (38.475, -4.2868) -> (38.327, -4.369)
  line L494 (38.327, -4.369) -> (38.1774, -4.4454)
  line L495 (38.1774, -4.4454) -> (38.1499, -4.4639)
  line L496 (38.1499, -4.4639) -> (38.1186, -4.4979)
  line L497 (38.1186, -4.4979) -> (38.0943, -4.5421)
  line L498 (38.0943, -4.5421) -> (38.0778, -4.596)
  line L499 (38.0778, -4.596) -> (38.0699, -4.659)
  line L500 (38.0699, -4.659) -> (38.0712, -4.7305)
  line L501 (38.0712, -4.7305) -> (38.0825, -4.8097)
  line L502 (38.0825, -4.8097) -> (38.1043, -4.896)
  line L503 (38.1043, -4.896) -> (38.1374, -4.9886)
  line L504 (38.1374, -4.9886) -> (38.1822, -5.0867)
  line L505 (38.1822, -5.0867) -> (38.2393, -5.1894)
  line L506 (38.2393, -5.1894) -> (38.2546, -5.238)
  line L507 (38.2546, -5.238) -> (38.2738, -5.3276)
  line L508 (38.2738, -5.3276) -> (38.2905, -5.4578)
  line L509 (38.2905, -5.4578) -> (38.2959, -5.5376)
  line L510 (38.2959, -5.5376) -> (38.2981, -5.6283)
  line L511 (38.2981, -5.6283) -> (38.2965, -5.7275)
  line L512 (38.2965, -5.7275) -> (38.2899, -5.8384)
  line L513 (38.2899, -5.8384) -> (38.278, -5.9569)
  line L514 (38.278, -5.9569) -> (38.2595, -6.0859)
  line L515 (38.2595, -6.0859) -> (38.2339, -6.2232)
  line L516 (38.2339, -6.2232) -> (38.2002, -6.3695)
  line L517 (38.2002, -6.3695) -> (38.1578, -6.5238)
  line L518 (38.1578, -6.5238) -> (38.1096, -6.6745)
  arc A13 (37.5103, -6.8351) -> (38.1096, -6.6745) centre (36, 0) ccw
  line L519 (37.5103, -6.8351) -> (37.3931, -6.7287)
  line L520 (37.3931, -6.7287) -> (37.2793, -6.6163)
  line L521 (37.2793, -6.6163) -> (37.177, -6.5064)
  line L522 (37.177, -6.5064) -> (37.0862, -6.4003)
  line L523 (37.0862, -6.4003) -> (37.0056, -6.2978)
  line L524 (37.0056, -6.2978) -> (36.9361, -6.2012)
  line L525 (36.9361, -6.2012) -> (36.875, -6.1084)
  line L526 (36.875, -6.1084) -> (36.8239, -6.0233)
  line L527 (36.8239, -6.0233) -> (36.7805, -5.9436)
  line L528 (36.7805, -5.9436) -> (36.7452, -5.8718)
  line L529 (36.7452, -5.8718) -> (36.6947, -5.7507)
  line L530 (36.6947, -5.7507) -> (36.6665, -5.6635)
  line L531 (36.6665, -5.6635) -> (36.6555, -5.6138)
  line L532 (36.6555, -5.6138) -> (36.6535, -5.4963)
  line L533 (36.6535, -5.4963) -> (36.6433, -5.389)
  line L534 (36.6433, -5.389) -> (36.6256, -5.2923)
  line L535 (36.6256, -5.2923) -> (36.6014, -5.2066)
  line L536 (36.6014, -5.2066) -> (36.5716, -5.1323)
  line L537 (36.5716, -5.1323) -> (36.537, -5.0698)
  line L538 (36.537, -5.0698) -> (36.4986, -5.0192)
  line L539 (36.4986, -5.0192) -> (36.4573, -4.9808)
  line L540 (36.4573, -4.9808) -> (36.4142, -4.9546)
  line L541 (36.4142, -4.9546) -> (36.3701, -4.9408)
  line L542 (36.3701, -4.9408) -> (36.337, -4.9386)
  line L543 (36.337, -4.9386) -> (36.1693, -4.9471)
  line L544 (36.1693, -4.9471) -> (36, -4.95)
  line L545 (36, -4.95) -> (35.8307, -4.9471)
  line L546 (35.8307, -4.9471) -> (35.663, -4.9386)
  line L547 (35.663, -4.9386) -> (35.6299, -4.9408)
  line L548 (35.6299, -4.9408) -> (35.5858, -4.9546)
  line L549 (35.5858, -4.9546) -> (35.5427, -4.9808)
  line L550 (35.5427, -4.9808) -> (35.5014, -5.0192)
  line L551 (35.5014, -5.0192) -> (35.463, -5.0698)
  line L552 (35.463, -5.0698) -> (35.4284, -5.1323)
  line L553 (35.4284, -5.1323) -> (35.3986, -5.2066)
  line L554 (35.3986, -5.2066) -> (35.3744, -5.2923)
  line L555 (35.3744, -5.2923) -> (35.3567, -5.389)
  line L556 (35.3567, -5.389) -> (35.3465, -5.4963)
  line L557 (35.3465, -5.4963) -> (35.3445, -5.6138)
  line L558 (35.3445, -5.6138) -> (35.3335, -5.6635)
  line L559 (35.3335, -5.6635) -> (35.3053, -5.7507)
  line L560 (35.3053, -5.7507) -> (35.2548, -5.8718)
  line L561 (35.2548, -5.8718) -> (35.2195, -5.9436)
  line L562 (35.2195, -5.9436) -> (35.1761, -6.0233)
  line L563 (35.1761, -6.0233) -> (35.125, -6.1084)
  line L564 (35.125, -6.1084) -> (35.0639, -6.2012)
  line L565 (35.0639, -6.2012) -> (34.9944, -6.2978)
  line L566 (34.9944, -6.2978) -> (34.9138, -6.4003)
  line L567 (34.9138, -6.4003) -> (34.823, -6.5064)
  line L568 (34.823, -6.5064) -> (34.7207, -6.6163)
  line L569 (34.7207, -6.6163) -> (34.6069, -6.7287)
  line L570 (34.6069, -6.7287) -> (34.4897, -6.8351)
  arc A14 (33.8904, -6.6745) -> (34.4897, -6.8351) centre (36, 0) ccw
  line L571 (33.8904, -6.6745) -> (33.8422, -6.5238)
  line L572 (33.8422, -6.5238) -> (33.7998, -6.3695)
  line L573 (33.7998, -6.3695) -> (33.7661, -6.2232)
  line L574 (33.7661, -6.2232) -> (33.7405, -6.0859)
  line L575 (33.7405, -6.0859) -> (33.722, -5.9569)
  line L576 (33.722, -5.9569) -> (33.7101, -5.8384)
  line L577 (33.7101, -5.8384) -> (33.7035, -5.7275)
  line L578 (33.7035, -5.7275) -> (33.7019, -5.6283)
  line L579 (33.7019, -5.6283) -> (33.7041, -5.5376)
  line L580 (33.7041, -5.5376) -> (33.7095, -5.4578)
  line L581 (33.7095, -5.4578) -> (33.7262, -5.3276)
  line L582 (33.7262, -5.3276) -> (33.7454, -5.238)
  line L583 (33.7454, -5.238) -> (33.7607, -5.1894)
  line L584 (33.7607, -5.1894) -> (33.8178, -5.0867)
  line L585 (33.8178, -5.0867) -> (33.8626, -4.9886)
  line L586 (33.8626, -4.9886) -> (33.8957, -4.896)
  line L587 (33.8957, -4.896) -> (33.9175, -4.8097)
  line L588 (33.9175, -4.8097) -> (33.9288, -4.7305)
  line L589 (33.9288, -4.7305) -> (33.9301, -4.659)
  line L590 (33.9301, -4.659) -> (33.9222, -4.596)
  line L591 (33.9222, -4.596) -> (33.9057, -4.5421)
  line L592 (33.9057, -4.5421) -> (33.8814, -4.4979)
  line L593 (33.8814, -4.4979) -> (33.8501, -4.4639)
  line L594 (33.8501, -4.4639) -> (33.8226, -4.4454)
  line L595 (33.8226, -4.4454) -> (33.673, -4.369)
  line L596 (33.673, -4.369) -> (33.525, -4.2868)
  line L597 (33.525, -4.2868) -> (33.3798, -4.1997)
  line L598 (33.3798, -4.1997) -> (33.2389, -4.1084)
  line L599 (33.2389, -4.1084) -> (33.2091, -4.0938)
  line L600 (33.2091, -4.0938) -> (33.164, -4.0837)
  line L601 (33.164, -4.0837) -> (33.1136, -4.0848)
  line L602 (33.1136, -4.0848) -> (33.0586, -4.0975)
  line L603 (33.0586, -4.0975) -> (33.0001, -4.1221)
  line L604 (33.0001, -4.1221) -> (32.9389, -4.159)
  line L605 (32.9389, -4.159) -> (32.8759, -4.2083)
  line L606 (32.8759, -4.2083) -> (32.8121, -4.2704)
  line L607 (32.8121, -4.2704) -> (32.7484, -4.3453)
  line L608 (32.7484, -4.3453) -> (32.6859, -4.4332)
  line L609 (32.6859, -4.4332) -> (32.6254, -4.534)
  line L610 (32.6254, -4.534) -> (32.5911, -4.5715)
  line L611 (32.5911, -4.5715) -> (32.523, -4.6329)
  line L612 (32.523, -4.6329) -> (32.4187, -4.7125)
  line L613 (32.4187, -4.7125) -> (32.3522, -4.7571)
  line L614 (32.3522, -4.7571) -> (32.2748, -4.8044)
  line L615 (32.2748, -4.8044) -> (32.1881, -4.8525)
  line L616 (32.1881, -4.8525) -> (32.0888, -4.9023)
  line L617 (32.0888, -4.9023) -> (31.9802, -4.9512)
  line L618 (31.9802, -4.9512) -> (31.8592, -4.9997)
  line L619 (31.8592, -4.9997) -> (31.7275, -5.0462)
  line L620 (31.7275, -5.0462) -> (31.5839, -5.0902)
  line L621 (31.5839, -5.0902) -> (31.4292, -5.1306)
  line L622 (31.4292, -5.1306) -> (31.2745, -5.1642)
  arc A15 (30.8358, -4.7255) -> (31.2745, -5.1642) centre (36, 0) ccw
  line L623 (30.8358, -4.7255) -> (30.8694, -4.5708)
  line L624 (30.676, 2.741) -> (30.453, 2.6211)
  line L625 (30.453, 2.6211) -> (30.2376, 2.5111)
  line L626 (30.2376, 2.5111) -> (30.0323, 2.4116)
  line L627 (30.0323, 2.4116) -> (29.8355, 2.3213)
  line L628 (29.8355, 2.3213) -> (29.6473, 2.2396)
  line L629 (29.6473, 2.2396) -> (29.4705, 2.1673)
  line L630 (29.4705, 2.1673) -> (29.3033, 2.1029)
  line L631 (29.3033, 2.1029) -> (28.9724, 1.9849)
  line L632 (28.9724, 1.9849) -> (28.931, 1.9629)
  line L633 (28.931, 1.9629) -> (28.9033, 1.9404)
  line L634 (28.9033, 1.9404) -> (28.8892, 1.9178)
  line L635 (28.8892, 1.9178) -> (28.8876, 1.9012)
  line L636 (28.8876, 1.9012) -> (28.9103, 1.5151)
  line L637 (28.9103, 1.5151) -> (28.9281, 1.1288)
  line L638 (28.9281, 1.1288) -> (28.9314, 1.1124)
  line L639 (28.9314, 1.1124) -> (28.9478, 1.0915)
  line L640 (28.9478, 1.0915) -> (28.9777, 1.0719)
  line L641 (28.9777, 1.0719) -> (29.0211, 1.0544)
  line L642 (29.0211, 1.0544) -> (29.3626, 0.9717)
  line L643 (29.3626, 0.9717) -> (29.5356, 0.9251)
  line L644 (29.5356, 0.9251) -> (29.719, 0.8717)
  line L645 (29.719, 0.8717) -> (29.9147, 0.8101)
  line L646 (29.9147, 0.8101) -> (30.1199, 0.7408)
  line L647 (30.1199, 0.7408) -> (30.3344, 0.6634)
  line L648 (30.3344, 0.6634) -> (30.5601, 0.5765)
  line L649 (30.5601, 0.5765) -> (30.7945, 0.4805)
  line L650 (30.7945, 0.4805) -> (30.9975, 0.3928)
  arc A16 (30.9975, -0.3928) -> (30.9975, 0.3928) centre (0, 0) ccw
  line L651 (30.9975, -0.3928) -> (30.7945, -0.4805)
  line L652 (30.7945, -0.4805) -> (30.5601, -0.5765)
  line L653 (30.5601, -0.5765) -> (30.3344, -0.6634)
  line L654 (30.3344, -0.6634) -> (30.1199, -0.7408)
  line L655 (30.1199, -0.7408) -> (29.9147, -0.8101)
  line L656 (29.9147, -0.8101) -> (29.719, -0.8717)
  line L657 (29.719, -0.8717) -> (29.5356, -0.9251)
  line L658 (29.5356, -0.9251) -> (29.3626, -0.9717)
  line L659 (29.3626, -0.9717) -> (29.0211, -1.0544)
  line L660 (29.0211, -1.0544) -> (28.9777, -1.0719)
  line L661 (28.9777, -1.0719) -> (28.9478, -1.0915)
  line L662 (28.9478, -1.0915) -> (28.9314, -1.1124)
  line L663 (28.9314, -1.1124) -> (28.9281, -1.1288)
  line L664 (28.9281, -1.1288) -> (28.9103, -1.5151)
  line L665 (28.9103, -1.5151) -> (28.8876, -1.9012)
  line L666 (28.8876, -1.9012) -> (28.8892, -1.9178)
  line L667 (28.8892, -1.9178) -> (28.9033, -1.9404)
  line L668 (28.9033, -1.9404) -> (28.931, -1.9629)
  line L669 (28.931, -1.9629) -> (28.9724, -1.9849)
  line L670 (28.9724, -1.9849) -> (29.3033, -2.1029)
  line L671 (29.3033, -2.1029) -> (29.4705, -2.1673)
  line L672 (29.4705, -2.1673) -> (29.6473, -2.2396)
  line L673 (29.6473, -2.2396) -> (29.8355, -2.3213)
  line L674 (29.8355, -2.3213) -> (30.0323, -2.4116)
  line L675 (30.0323, -2.4116) -> (30.2376, -2.5111)
  line L676 (30.2376, -2.5111) -> (30.453, -2.6211)
  line L677 (30.453, -2.6211) -> (30.676, -2.741)
  line L678 (30.676, -2.741) -> (30.8688, -2.8495)
  arc A17 (30.7866, -3.6308) -> (30.8688, -2.8495) centre (0, 0) ccw
  line L679 (30.7866, -3.6308) -> (30.5755, -3.6968)
  line L680 (30.5755, -3.6968) -> (30.3325, -3.7677)
  line L681 (30.3325, -3.7677) -> (30.0989, -3.8305)
  line L682 (30.0989, -3.8305) -> (29.8774, -3.8852)
  line L683 (29.8774, -3.8852) -> (29.6661, -3.9326)
  line L684 (29.6661, -3.9326) -> (29.465, -3.9734)
  line L685 (29.465, -3.9734) -> (29.2771, -4.0074)
  line L686 (29.2771, -4.0074) -> (29.1001, -4.0356)
  line L687 (29.1001, -4.0356) -> (28.7519, -4.0822)
  line L688 (28.7519, -4.0822) -> (28.7069, -4.0951)
  line L689 (28.7069, -4.0951) -> (28.6751, -4.1114)
  line L690 (28.6751, -4.1114) -> (28.6567, -4.1305)
  line L691 (28.6567, -4.1305) -> (28.6516, -4.1464)
  line L692 (28.6516, -4.1464) -> (28.5936, -4.5288)
  line L693 (28.5936, -4.5288) -> (28.5306, -4.9104)
  line L694 (28.5306, -4.9104) -> (28.5305, -4.927)
  line L695 (28.5305, -4.927) -> (28.5421, -4.951)
  line L696 (28.5421, -4.951) -> (28.5674, -4.9763)
  line L697 (28.5674, -4.9763) -> (28.6062, -5.0025)
  line L698 (28.6062, -5.0025) -> (28.9229, -5.1544)
  line L699 (28.9229, -5.1544) -> (29.0826, -5.2359)
  line L700 (29.0826, -5.2359) -> (29.2508, -5.3263)
  line L701 (29.2508, -5.3263) -> (29.4294, -5.4272)
  line L702 (29.4294, -5.4272) -> (29.6157, -5.5376)
  line L703 (29.6157, -5.5376) -> (29.8094, -5.658)
  line L704 (29.8094, -5.658) -> (30.0122, -5.79)
  line L705 (30.0122, -5.79) -> (30.2214, -5.9325)
  line L706 (30.2214, -5.9325) -> (30.4018, -6.0605)
  arc A18 (30.2385, -6.829) -> (30.4018, -6.0605) centre (0, 0) ccw
  line L707 (30.2385, -6.829) -> (30.0216, -6.8726)
  line L708 (30.0216, -6.8726) -> (29.7725, -6.9177)
  line L709 (29.7725, -6.9177) -> (29.5336, -6.9557)
  line L710 (29.5336, -6.9557) -> (29.3077, -6.9869)
  line L711 (29.3077, -6.9869) -> (29.0926, -7.012)
  line L712 (29.0926, -7.012) -> (28.8883, -7.0315)
  line L713 (28.8883, -7.0315) -> (28.6979, -7.0457)
  line L714 (28.6979, -7.0457) -> (28.5189, -7.0553)
  line L715 (28.5189, -7.0553) -> (28.1677, -7.0652)
  line L716 (28.1677, -7.0652) -> (28.1216, -7.0733)
  line L717 (28.1216, -7.0733) -> (28.0883, -7.0862)
  line L718 (28.0883, -7.0862) -> (28.0679, -7.1033)
  line L719 (28.0679, -7.1033) -> (28.0612, -7.1186)
  line L720 (28.0612, -7.1186) -> (27.9636, -7.4928)
  line L721 (27.9636, -7.4928) -> (27.861, -7.8657)
  line L722 (27.861, -7.8657) -> (27.8592, -7.8823)
  line L723 (27.8592, -7.8823) -> (27.8683, -7.9073)
  line L724 (27.8683, -7.9073) -> (27.8907, -7.9351)
  line L725 (27.8907, -7.9351) -> (27.9266, -7.9652)
  line L726 (27.9266, -7.9652) -> (28.2257, -8.1494)
  line L727 (28.2257, -8.1494) -> (28.3759, -8.2472)
  line L728 (28.3759, -8.2472) -> (28.5338, -8.3547)
  line L729 (28.5338, -8.3547) -> (28.7009, -8.4737)
  line L730 (28.7009, -8.4737) -> (28.8746, -8.603)
  line L731 (28.8746, -8.603) -> (29.0547, -8.7429)
  line L732 (29.0547, -8.7429) -> (29.2425, -8.8954)
  line L733 (29.2425, -8.8954) -> (29.4358, -9.059)
  line L734 (29.4358, -9.059) -> (29.6018, -9.2052)
  arc A19 (29.359, -9.9523) -> (29.6018, -9.2052) centre (0, 0) ccw
  line L735 (29.359, -9.9523) -> (29.1388, -9.973)
  line L736 (29.1388, -9.973) -> (28.8863, -9.9918)
  line L737 (28.8863, -9.9918) -> (28.6447, -10.0047)
  line L738 (28.6447, -10.0047) -> (28.4168, -10.0121)
  line L739 (28.4168, -10.0121) -> (28.2002, -10.0146)
  line L740 (28.2002, -10.0146) -> (27.995, -10.0127)
  line L741 (27.995, -10.0127) -> (27.8042, -10.0069)
  line L742 (27.8042, -10.0069) -> (27.6252, -9.9977)
  line L743 (27.6252, -9.9977) -> (27.2749, -9.9708)
  line L744 (27.2749, -9.9708) -> (27.2282, -9.9741)
  line L745 (27.2282, -9.9741) -> (27.1937, -9.9834)
  line L746 (27.1937, -9.9834) -> (27.1717, -9.9983)
  line L747 (27.1717, -9.9983) -> (27.1634, -10.0128)
  line L748 (27.1634, -10.0128) -> (27.0272, -10.3748)
  line L749 (27.0272, -10.3748) -> (26.8862, -10.7349)
  line L750 (26.8862, -10.7349) -> (26.8826, -10.7512)
  line L751 (26.8826, -10.7512) -> (26.8891, -10.777)
  line L752 (26.8891, -10.777) -> (26.9085, -10.807)
  line L753 (26.9085, -10.807) -> (26.941, -10.8407)
  line L754 (26.941, -10.8407) -> (27.2193, -11.0551)
  line L755 (27.2193, -11.0551) -> (27.3584, -11.1681)
  line L756 (27.3584, -11.1681) -> (27.5042, -11.2915)
  line L757 (27.5042, -11.2915) -> (27.6579, -11.4273)
  line L758 (27.6579, -11.4273) -> (27.8172, -11.5741)
  line L759 (27.8172, -11.5741) -> (27.9817, -11.7321)
  line L760 (27.9817, -11.7321) -> (28.1525, -11.9033)
  line L761 (28.1525, -11.9033) -> (28.3276, -12.0862)
  line L762 (28.3276, -12.0862) -> (28.4774, -12.249)
  arc A20 (28.1579, -12.9667) -> (28.4774, -12.249) centre (0, 0) ccw
  line L763 (28.1579, -12.9667) -> (27.9367, -12.9642)
  line L764 (27.9367, -12.9642) -> (27.6836, -12.9565)
  line L765 (27.6836, -12.9565) -> (27.442, -12.9441)
  line L766 (27.442, -12.9441) -> (27.2145, -12.9276)
  line L767 (27.2145, -12.9276) -> (26.9989, -12.9075)
  line L768 (26.9989, -12.9075) -> (26.7951, -12.8841)
  line L769 (26.7951, -12.8841) -> (26.6059, -12.8584)
  line L770 (26.6059, -12.8584) -> (26.4288, -12.8305)
  line L771 (26.4288, -12.8305) -> (26.0833, -12.7672)
  line L772 (26.0833, -12.7672) -> (26.0365, -12.7656)
  line L773 (26.0365, -12.7656) -> (26.0012, -12.7712)
  line L774 (26.0012, -12.7712) -> (25.9777, -12.7837)
  line L775 (25.9777, -12.7837) -> (25.968, -12.7973)
  line L776 (25.968, -12.7973) -> (25.7946, -13.143)
  line L777 (25.7946, -13.143) -> (25.6168, -13.4865)
  line L778 (25.6168, -13.4865) -> (25.6116, -13.5023)
  line L779 (25.6116, -13.5023) -> (25.6153, -13.5287)
  line L780 (25.6153, -13.5287) -> (25.6314, -13.5605)
  line L781 (25.6314, -13.5605) -> (25.6603, -13.5974)
  line L782 (25.6603, -13.5974) -> (25.9146, -13.8398)
  line L783 (25.9146, -13.8398) -> (26.0412, -13.9666)
  line L784 (26.0412, -13.9666) -> (26.1732, -14.1046)
  line L785 (26.1732, -14.1046) -> (26.312, -14.2558)
  line L786 (26.312, -14.2558) -> (26.455, -14.4184)
  line L787 (26.455, -14.4184) -> (26.602, -14.5927)
  line L788 (26.602, -14.5927) -> (26.7541, -14.7808)
  line L789 (26.7541, -14.7808) -> (26.9091, -14.9811)
  line L790 (26.9091, -14.9811) -> (27.041, -15.1586)
  arc A21 (26.6482, -15.8389) -> (27.041, -15.1586) centre (0, 0) ccw
  line L791 (26.6482, -15.8389) -> (26.4285, -15.8134)
  line L792 (26.4285, -15.8134) -> (26.1776, -15.7793)
  line L793 (26.1776, -15.7793) -> (25.9387, -15.7417)
  line L794 (25.9387, -15.7417) -> (25.7142, -15.7015)
  line L795 (25.7142, -15.7015) -> (25.5018, -15.6589)
  line L796 (25.5018, -15.6589) -> (25.3015, -15.6144)
  line L797 (25.3015, -15.6144) -> (25.1161, -15.569)
  line L798 (25.1161, -15.569) -> (24.9429, -15.5228)
  line L799 (24.9429, -15.5228) -> (24.6058, -15.4237)
  line L800 (24.6058, -15.4237) -> (24.5595, -15.4172)
  line L801 (24.5595, -15.4172) -> (24.5238, -15.4191)
  line L802 (24.5238, -15.4191) -> (24.4991, -15.4291)
  line L803 (24.4991, -15.4291) -> (24.488, -15.4416)
  line L804 (24.488, -15.4416) -> (24.2795, -15.7673)
  line L805 (24.2795, -15.7673) -> (24.0668, -16.0903)
  line L806 (24.0668, -16.0903) -> (24.0599, -16.1055)
  line L807 (24.0599, -16.1055) -> (24.0608, -16.1321)
  line L808 (24.0608, -16.1321) -> (24.0735, -16.1655)
  line L809 (24.0735, -16.1655) -> (24.0984, -16.2052)
  line L810 (24.0984, -16.2052) -> (24.326, -16.4728)
  line L811 (24.326, -16.4728) -> (24.4386, -16.6122)
  line L812 (24.4386, -16.6122) -> (24.5555, -16.7632)
  line L813 (24.5555, -16.7632) -> (24.6777, -16.928)
  line L814 (24.6777, -16.928) -> (24.8029, -17.1047)
  line L815 (24.8029, -17.1047) -> (24.931, -17.2934)
  line L816 (24.931, -17.2934) -> (25.0625, -17.4964)
  line L817 (25.0625, -17.4964) -> (25.1957, -17.7118)
  line L818 (25.1957, -17.7118) -> (25.3084, -17.9021)
  arc A22 (24.8466, -18.5377) -> (25.3084, -17.9021) centre (0, 0) ccw
  line L819 (24.8466, -18.5377) -> (24.6308, -18.4893)
  line L820 (24.6308, -18.4893) -> (24.3848, -18.4292)
  line L821 (24.3848, -18.4292) -> (24.1511, -18.3668)
  line L822 (24.1511, -18.3668) -> (23.932, -18.3034)
  line L823 (23.932, -18.3034) -> (23.7253, -18.2388)
  line L824 (23.7253, -18.2388) -> (23.5308, -18.1736)
  line L825 (23.5308, -18.1736) -> (23.3511, -18.1091)
  line L826 (23.3511, -18.1091) -> (23.1837, -18.045)
  line L827 (23.1837, -18.045) -> (22.8588, -17.9112)
  line L828 (22.8588, -17.9112) -> (22.8134, -17.8999)
  line L829 (22.8134, -17.8999) -> (22.7777, -17.8981)
  line L830 (22.7777, -17.8981) -> (22.7521, -17.9055)
  line L831 (22.7521, -17.9055) -> (22.7398, -17.9167)
  line L832 (22.7398, -17.9167) -> (22.4984, -18.2188)
  line L833 (22.4984, -18.2188) -> (22.2531, -18.5178)
  line L834 (22.2531, -18.5178) -> (22.2446, -18.5322)
  line L835 (22.2446, -18.5322) -> (22.2427, -18.5587)
  line L836 (22.2427, -18.5587) -> (22.2519, -18.5933)
  line L837 (22.2519, -18.5933) -> (22.2724, -18.6353)
  line L838 (22.2724, -18.6353) -> (22.4708, -18.9253)
  line L839 (22.4708, -18.9253) -> (22.5683, -19.0757)
  line L840 (22.5683, -19.0757) -> (22.6688, -19.2381)
  line L841 (22.6688, -19.2381) -> (22.773, -19.4148)
  line L842 (22.773, -19.4148) -> (22.8791, -19.6036)
  line L843 (22.8791, -19.6036) -> (22.9867, -19.8047)
  line L844 (22.9867, -19.8047) -> (23.0963, -20.0203)
  line L845 (23.0963, -20.0203) -> (23.2063, -20.2484)
  line L846 (23.2063, -20.2484) -> (23.2985, -20.4495)
  arc A23 (22.7728, -21.0333) -> (23.2985, -20.4495) centre (0, 0) ccw
  line L847 (22.7728, -21.0333) -> (22.5632, -20.9626)
  line L848 (22.5632, -20.9626) -> (22.3249, -20.8771)
  line L849 (22.3249, -20.8771) -> (22.099, -20.7906)
  line L850 (22.099, -20.7906) -> (21.8877, -20.7047)
  line L851 (21.8877, -20.7047) -> (21.6889, -20.6189)
  line L852 (21.6889, -20.6189) -> (21.5022, -20.5336)
  line L853 (21.5022, -20.5336) -> (21.3302, -20.4507)
  line L854 (21.3302, -20.4507) -> (21.1705, -20.3695)
  line L855 (21.1705, -20.3695) -> (20.8614, -20.2025)
  line L856 (20.8614, -20.2025) -> (20.8174, -20.1865)
  line L857 (20.8174, -20.1865) -> (20.7821, -20.181)
  line L858 (20.7821, -20.181) -> (20.7559, -20.1856)
  line L859 (20.7559, -20.1856) -> (20.7424, -20.1955)
  line L860 (20.7424, -20.1955) -> (20.4707, -20.4707)
  line L861 (20.4707, -20.4707) -> (20.1955, -20.7424)
  line L862 (20.1955, -20.7424) -> (20.1856, -20.7559)
  line L863 (20.1856, -20.7559) -> (20.181, -20.7821)
  line L864 (20.181, -20.7821) -> (20.1865, -20.8174)
  line L865 (20.1865, -20.8174) -> (20.2025, -20.8614)
  line L866 (20.2025, -20.8614) -> (20.3695, -21.1705)
  line L867 (20.3695, -21.1705) -> (20.4507, -21.3302)
  line L868 (20.4507, -21.3302) -> (20.5336, -21.5022)
  line L869 (20.5336, -21.5022) -> (20.6189, -21.6889)
  line L870 (20.6189, -21.6889) -> (20.7047, -21.8877)
  line L871 (20.7047, -21.8877) -> (20.7906, -22.099)
  line L872 (20.7906, -22.099) -> (20.8771, -22.3249)
  line L873 (20.8771, -22.3249) -> (20.9626, -22.5632)
  line L874 (20.9626, -22.5632) -> (21.0333, -22.7728)
  arc A24 (20.4495, -23.2985) -> (21.0333, -22.7728) centre (0, 0) ccw
  line L875 (20.4495, -23.2985) -> (20.2484, -23.2063)
  line L876 (20.2484, -23.2063) -> (20.0203, -23.0963)
  line L877 (20.0203, -23.0963) -> (19.8047, -22.9867)
  line L878 (19.8047, -22.9867) -> (19.6036, -22.8791)
  line L879 (19.6036, -22.8791) -> (19.4148, -22.773)
  line L880 (19.4148, -22.773) -> (19.2381, -22.6688)
  line L881 (19.2381, -22.6688) -> (19.0757, -22.5683)
  line L882 (19.0757, -22.5683) -> (18.9253, -22.4708)
  line L883 (18.9253, -22.4708) -> (18.6353, -22.2724)
  line L884 (18.6353, -22.2724) -> (18.5933, -22.2519)
  line L885 (18.5933, -22.2519) -> (18.5587, -22.2427)
  line L886 (18.5587, -22.2427) -> (18.5322, -22.2446)
  line L887 (18.5322, -22.2446) -> (18.5178, -22.2531)
  line L888 (18.5178, -22.2531) -> (18.2188, -22.4984)
  line L889 (18.2188, -22.4984) -> (17.9167, -22.7398)
  line L890 (17.9167, -22.7398) -> (17.9055, -22.7521)
  line L891 (17.9055, -22.7521) -> (17.8981, -22.7777)
  line L892 (17.8981, -22.7777) -> (17.8999, -22.8134)
  line L893 (17.8999, -22.8134) -> (17.9112, -22.8588)
  line L894 (17.9112, -22.8588) -> (18.045, -23.1837)
  line L895 (18.045, -23.1837) -> (18.1091, -23.3511)
  line L896 (18.1091, -23.3511) -> (18.1736, -23.5308)
  line L897 (18.1736, -23.5308) -> (18.2388, -23.7253)
  line L898 (18.2388, -23.7253) -> (18.3034, -23.932)
  line L899 (18.3034, -23.932) -> (18.3668, -24.1511)
  line L900 (18.3668, -24.1511) -> (18.4292, -24.3848)
  line L901 (18.4292, -24.3848) -> (18.4893, -24.6308)
  line L902 (18.4893, -24.6308) -> (18.5377, -24.8466)
  arc A25 (17.9021, -25.3084) -> (18.5377, -24.8466) centre (0, 0) ccw
  line L903 (17.9021, -25.3084) -> (17.7118, -25.1957)
  line L904 (17.7118, -25.1957) -> (17.4964, -25.0625)
  line L905 (17.4964, -25.0625) -> (17.2934, -24.931)
  line L906 (17.2934, -24.931) -> (17.1047, -24.8029)
  line L907 (17.1047, -24.8029) -> (16.928, -24.6777)
  line L908 (16.928, -24.6777) -> (16.7632, -24.5555)
  line L909 (16.7632, -24.5555) -> (16.6122, -24.4386)
  line L910 (16.6122, -24.4386) -> (16.4728, -24.326)
  line L911 (16.4728, -24.326) -> (16.2052, -24.0984)
  line L912 (16.2052, -24.0984) -> (16.1655, -24.0735)
  line L913 (16.1655, -24.0735) -> (16.1321, -24.0608)
  line L914 (16.1321, -24.0608) -> (16.1055, -24.0599)